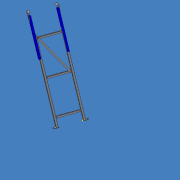
# Autodesk Inventor part: 90-08-1550
Saved by Autodesk Inventor 2015 SP1 (Build 190203100, 203)
## iProperties
Created: 2007-08-02
Part Number: 90-08-1550
Material: Steel, Mild
Document SubType Name: Modeling
Designer: kurt
Manufacturer: Standard
Standards Organization: Custom
Density: 7.86 g/cm^3
Appearance: Steel
Behandeling: Behandeling
Besteld: S
Materiaal: st37
Totaal: 0
Author: kurt
Autodesk Inventor part; units mm, degrees
ref_plane "YZ Plane" through (0, 0, 0) normal (1, 0, 0) x (0, 1, 0)
ref_plane "XZ Plane" through (0, 0, 0) normal (0, 1, 0) x (-1, 0, 0)
ref_plane "XY Plane" through (0, 0, 0) normal (0, 0, 1) x (1, 0, 0)
sketch "Sketch1" plane through (0, 0, 0) normal (0, 0, 1) x (1, 0, 0)
  circle A0 centre (190, 3.5) radius 5.5 projected
  circle A1 centre (-192, 668.25) radius 5.5 projected
  arc A2 (176.9945, -3.9737) -> (203.0055, 10.9737) centre (190, 3.5) ccw
  arc A3 (-178.9945, 675.7237) -> (-205.0055, 660.7763) centre (-192, 668.25) ccw
  circle A4 centre (190, 3.5) radius 5.5
  circle A5 centre (-192, 668.25) radius 5.5
  line L0 (-178.9945, 675.7237) -> (203.0055, 10.9737)
  line L1 (176.9945, -3.9737) -> (-205.0055, 660.7763)
  point P0 (0, 0)
  dimension "d2" = 11
  dimension "d3" = 30
  dimension "d4" = 11
  dimension "d5" = 30
  constraints: 4 centre point, 4 coincident, 4 end point, 4 point on circle, 4 tangent
  measures "d2" diameter of A5
  measures "d3" diameter of A3
  measures "d4" diameter of A4
  measures "d5" diameter of A2
extrude "Extrusion2" add sketch "Sketch1" along normal blind 6
body "Solid1"
